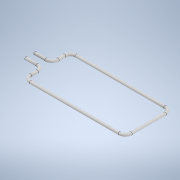
# Autodesk Inventor part: AC_heater_coil
Saved by Autodesk Inventor 2020 (Build 240168000, 168)
## iProperties
Created: 2022-09-01
Part Number: AC_heater_coil
Material: Generic
Document SubType Name: Modeling
Designer: Intuito_PC
Density: 1 g/cm^3
Appearance: Default
Author: Intuito_PC
Autodesk Inventor part; units mm, degrees
ref_plane "YZ Plane" through (0, 0, 0) normal (1, 0, 0) x (0, 1, 0)
ref_plane "XZ Plane" through (0, 0, 0) normal (0, 1, 0) x (-1, 0, 0)
sketch "Sketch1" plane through (0, 0, 0) normal (0, 1, 0) x (-1, 0, 0)
  line L0 (-234.6, -100) -> (154.7391, -100)
  line L1 (154.7391, 100) -> (-234.6, 100)
  line L2 (-260, 74.6) -> (-260, -74.6)
  line L3 (-260, -100) -> (260, 100) construction
  line L4 (260, -100) -> (-260, 100) construction
  line L5 (205.5391, 19.7022) -> (254.4067, 19.7022)
  line L6 (254.4067, -19.3359) -> (205.5391, -19.3359)
  line L7 (180.1391, 74.6) -> (180.1391, 45.1022)
  line L8 (180.1391, -44.7359) -> (180.1391, -74.6)
  arc A0 (180.1391, 74.6) -> (154.7391, 100) centre (154.7391, 74.6) ccw
  arc A1 (180.1391, 45.1022) -> (205.5391, 19.7022) centre (205.5391, 45.1022) ccw
  arc A2 (205.5391, -19.3359) -> (180.1391, -44.7359) centre (205.5391, -44.7359) ccw
  arc A3 (154.7391, -100) -> (180.1391, -74.6) centre (154.7391, -74.6) ccw
  arc A4 (-260, -74.6) -> (-234.6, -100) centre (-234.6, -74.6) ccw
  arc A5 (-234.6, 100) -> (-260, 74.6) centre (-234.6, 74.6) ccw
  point P0 (0, 0)
  dimension "d0" = 520
  dimension "d2" = 200
  dimension "d3" = 25.4
  dimension "d4" = 25.4
  constraints: 18 end point, 12 point on circle, 12 tangent, 6 centre point, 4 equal radius, 4 point on line, 2 horizontal, 2 midpoint, 2 parallel, 2 perpendicular
  measures "d0" distance of L4.end L3.end
  measures "d2" distance of L4.end L3.start
  measures "d3" radius of A0
  measures "d4" radius of A5
ref_plane "Work Plane1" through (-254.4067, 0, 19.7022) normal (-1, 0, 0) x (0, -1, 0)
sketch "Sketch2" plane through (-254.4067, 0, 19.7022) normal (-1, 0, 0) x (0, -1, 0)
  circle A0 centre (0, 0) radius 6
  point P0 (0, -19.7022)
  dimension "d5" = 12
  constraints: 1 centre point
  measures "d5" diameter of A0
sweep "Sweep1" add profiles "Sketch2" path "Sketch1"
body "Solid1"
